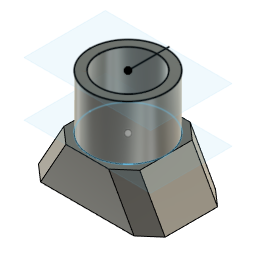
3350to32 (Autodesk Fusion 360 design; units mm, degrees)
Autodesk Fusion 360 part; units mm, degrees
sketch "草图1" plane through (0, 0, 0) normal (0, 1, 0) x (1, 0, 0)
  line L0 (0, 0) -> (70, 0)
  line L1 (70, 0) -> (70, -55)
  line L2 (70, -55) -> (0, -55)
  line L3 (0, -55) -> (0, 0)
  dimension "d1" = 70
  dimension "d2" = 55
  constraint horizontal L0
  constraint vertical L1
  constraint horizontal L2
  constraint vertical L3
  constraint coincident L0.start L3.end
  measures "d1" distance of L0.start L0.end
  measures "d2" distance of L0.start L2.end
extrude "拉伸1" add sketch "草图1" along normal blind 45
sketch "草图2" plane through (0, 0, 55) normal (0, 0, 1) x (-1, 0, 0)
  line L0 (0, 0) -> (-70, 0)
  line L1 (-70, 0) -> (-70, -45)
  line L2 (-70, -45) -> (0, -45)
  line L3 (0, -45) -> (0, 0)
  line L4 (-35, -45) -> (-35, -22.5)
  circle A0 centre (-35, -22.5) radius 16
  circle A1 centre (-35, -22.5) radius 21
  dimension "d5" = 22.5
  dimension "d6" = 32
  dimension "d12" = 42
  constraint midpoint L2 L4.start
  constraint perpendicular L2 L4
  constraint coincident L4.end A0.centre
  constraint concentric A0 A1
  measures "d5" distance of L4.start L4.end
  measures "d6" diameter of A0
  measures "d12" diameter of A1
extrude "拉伸2" cut sketch "草图2" against normal blind 40 contours A0
sketch "草图3" plane through (0, 0, 0) normal (0, 0, -1) x (1, 0, 0)
  line L0 (70, 0) -> (0, 0)
  line L1 (0, 0) -> (0, -45)
  line L2 (0, -45) -> (70, -45)
  line L3 (70, -45) -> (70, 0)
  line L4 (35, 0) -> (35, -22.5)
  line L5 (60, -39) -> (10, -39)
  line L6 (10, -39) -> (10, -6)
  line L7 (10, -6) -> (60, -6)
  line L8 (60, -6) -> (60, -39)
  line L9 (60, -39) -> (10, -6) construction
  line L10 (10, -39) -> (60, -6) construction
  point P0 (35, -22.5)
  dimension "d9" = 22.5
  dimension "d10" = 50
  dimension "d11" = 33
  constraint midpoint L0 L4.start
  constraint perpendicular L0 L4
  constraint horizontal L5
  constraint perpendicular L5 L6
  constraint parallel L5 L7
  constraint parallel L6 L8
  constraint coincident L9 P0
  constraint coincident L10 P0
  constraint coincident P0 L4.end
  measures "d9" distance of L4.start P0
  measures "d10" distance of L6.end L7.end
  measures "d11" distance of L5.end L6.end
sketch "草图4" plane through (0, 0, 15) normal (0, 0, 1) x (-1, 0, 0)
  circle A0 centre (-35, -22.5) radius 16
loft "放样1" cut profiles "草图4", "草图3" section 1 section 2 contours L5 L6 L7 L8
extrude "拉伸4" cut sketch "草图2" against normal blind 30 contours L0 L1 L2 L3
sketch "草图5" plane through (0, 0, 25) normal (0, 0, 1) x (-1, 0, 0)
  circle A0 centre (-35, -22.5) radius 21
  line L0 (0, -45) -> (0, 0)
  line L1 (0, 0) -> (-70, 0)
  line L2 (-70, 0) -> (-70, -45)
  line L3 (-70, -45) -> (0, -45)
  circle A1 centre (-35, -22.5) radius 21
  constraint concentric A0 A1
sketch "草图6" plane through (0, 45, 0) normal (0, 1, 0) x (-1, 0, 0)
  line L0 (0, 25) -> (-70, 25)
  line L1 (-70, 25) -> (-70, 0)
  line L2 (-70, 0) -> (0, 0)
  line L3 (0, 0) -> (0, 25)
  line L4 (-35, 25) -> (-56, 25)
  line L5 (-56, 25) -> (-70, 0)
  line L6 (-35, 25) -> (-14, 25)
  line L7 (-14, 25) -> (0, 0)
  dimension "d17" = 21
  dimension "d18" = 21
  constraint midpoint L0 L4.start
  constraint parallel L0 L4
  constraint coincident L1.end L2.start
  constraint parallel L0 L6
  constraint coincident L2.end L3.start
  measures "d17" distance of L4.start L4.end
  measures "d18" distance of L4.start L6.end
extrude "拉伸5" cut sketch "草图6" against normal blind 45 contours L0 L3 L7 | L0 L1 L5
chamfer "倒角1" distance 8 angle 45 4 edges at (7, 45, 12.5) (7, 0, 12.5) (63, 45, 12.5) (63, 0, 12.5)
extrude "拉伸3" [suppressed]
